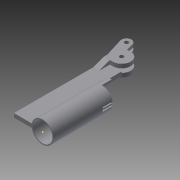
# Autodesk Inventor part: Base_Cylinder_1
Saved by Autodesk Inventor 2015 (Build 190159000, 159)
## iProperties
Created: 2016-07-06
Part Number: Base_Cylinder_1
Material: Generic
Document SubType Name: Modeling
Designer: Neelotpal Nag
Density: 1 g/cm^3
Appearance: Default
Mass: 1.76913 g
Surface Area: 37.308 cm^2
Volume: 1.76913 cm^3
Author: Neelotpal Nag
Autodesk Inventor part; units mm, degrees
ref_plane "YZ Plane" through (0, 0, 0) normal (1, 0, 0) x (0, 1, 0)
ref_plane "XZ Plane" through (0, 0, 0) normal (0, 1, 0) x (-1, 0, 0)
sketch "Sketch1" plane through (0, 0, 0) normal (0, 1, 0) x (-1, 0, 0)
  circle A0 centre (0, 0) radius 5
  circle A1 centre (0, 0) radius 5.5
  dimension "d0" = 10
  dimension "d1" = 11
  constraints: 2 centre point, 2 coincident
  measures "d0" diameter of A0
  measures "d1" diameter of A1
extrude "Extrusion1" add sketch "Sketch1" along normal blind 35
sketch "Sketch2" plane through (0, 0, 0) normal (0, 0, 1) x (1, 0, 0)
  point P0 (0, 0)
sketch "Sketch3" plane through (0, 0, 0) normal (0, 0, 1) x (1, 0, 0)
  line L0 (0, 0) -> (-10, 0)
  line L1 (-5.5, 0) -> (5.5, 0) projected
  circle A0 centre (-10, 50) radius 1
  line L2 (-5.5495, 50) -> (-5.5, 50)
  line L3 (-5.5, 50) -> (-5.5, 35)
  line L4 (5.5, 35) -> (-5.5, 35) projected
  line L5 (-14.5, 50) -> (-14.5, 0)
  line L6 (-14.5, 0) -> (-10, 0)
  circle A1 centre (-10, 50) radius 4.5
  line L7 (-10, 45.5) -> (-5.5, 45.5)
  line L8 (-14.5, 45.5) -> (-10, 45.5)
  line L9 (-5.5, 0) -> (-5.5, 50)
  line L10 (-5.5, 0) -> (-5.5, 45.5)
  line L11 (5, 0) -> (-5, 0) projected
  line L12 (-5.5, 0) -> (-5.5, 45.5)
  line L13 (-10, 0) -> (-5, 0)
  line L14 (-5.5, 45.5) -> (-5, 0)
  line L15 (-10, 0) -> (-10, 45.5)
  line L16 (-10, 45.5) -> (-5.5, 45.5)
  line L17 (-9, 50) -> (-10, 50)
  line L18 (-11, 50) -> (-14.5, 50)
  line L19 (-10, 0) -> (-10, 45.5)
  line L20 (-10, 49) -> (-10, 50)
  circle A2 centre (-10, 50) radius 4.5
  line L21 (-14.5, 45.5) -> (-14.5, 50)
  line L22 (-14.5, 45.5) -> (-5.5, 45.5)
  line L23 (-5.5, 45.5) -> (-5.5, 50)
  line L24 (-10, 50) -> (0, 50) construction
  line L25 (-10, 50) -> (-10.5736, 50.8192)
  circle A3 centre (-15.7358, 58.1915) radius 1
  circle A4 centre (-15.7358, 58.1915) radius 2.5
  point P0 (12.8857, 32.907)
  dimension "d4" = 10
  dimension "d5" = 50
  dimension "d7" = 2
  dimension "d8" = 9
  dimension "d19" = 2
  dimension "d20" = 5
  constraints: 47 end point, 8 collinear, 8 perpendicular, 7 coincident, 6 point on circle, 6 tangent, 5 centre point, 5 point on line, 2 horizontal, 2 vertical, 1 concentric
  measures "d4" distance of L0.start L0.end
  measures "d5" distance of L0.end L17.end
  measures "d7" diameter of A0
  measures "d8" distance of L2.end L5.start
  measures "d19" diameter of A3
  measures "d20" diameter of A4
extrude "Extrusion2" add sketch "Sketch3" along normal mid plane 2 contours L0 L9 L4 L14 | L0 L15 L7 L3 L9 | L4 L3 L14 | L6 L5 L8 L15
sketch "Sketch4" plane through (0, 0, 1) normal (0, 0, 1) x (1, 0, 0)
  circle A0 centre (-10, 50) radius 4.5 projected
  line L0 (-14.5, 50) -> (-14.5, 0) projected
  line L1 (-5.5, 50) -> (-5.5, 35) projected
  line L2 (-5.5, 45.5) -> (-14.5, 45.5) projected
  arc A1 (-14.5, 50) -> (-10, 45.5) centre (-10, 50) ccw
  line L3 (-10, 45.5) -> (-14.5, 45.5)
  line L4 (-14.5, 45.5) -> (-14.5, 50)
  point P0 (0, 0)
  constraints: 4 end point, 3 tangent, 2 point on circle, 1 centre point, 1 collinear, 1 concentric, 1 midpoint, 1 perpendicular
extrude "Extrusion3" add sketch "Sketch4" along normal blind 2 contours A0 L2 L0
sketch "Sketch5" plane through (0, 0, 1) normal (0, 0, 1) x (1, 0, 0)
  line L0 (-5.3846, 35) -> (-5.5, 45.5) projected
  line L1 (-5.4396, 40) -> (-14.5, 40)
  line L2 (-14.5, 45.5) -> (-14.5, 0) projected
  point P0 (0, 0)
  constraints: 2 end point, 2 point on line, 1 horizontal
sketch "Sketch6" plane through (-14.5, 45.5, 1) normal (-1, 0, 0) x (0, 0, 1)
  line L0 (2, 0) -> (0, -5.25)
  line L1 (0, -10.5) -> (0, 0) projected
  line L2 (2, 0) -> (0, 0)
  line L3 (0, 0) -> (0, -5.25)
  point P0 (-1, -45.5)
  constraints: 6 end point, 1 collinear, 1 horizontal, 1 midpoint
extrude "Extrusion4" add sketch "Sketch6" against normal blind 3
sketch "Sketch7" plane through (0, 0, 3) normal (0, 0, 1) x (1, 0, 0)
  circle A0 centre (-10, 50) radius 4.5 projected
  circle A1 centre (-10, 50) radius 1 projected
  point P0 (0, 0)
extrude "Extrusion5" add sketch "Sketch7" against normal blind 2
mirror "Mirror1" about plane through (0, 0, 0) normal (0, 0, 1) of "Extrusion4", "Extrusion3", "Extrusion5"
ref_plane "Work Plane1" through (0, 0, 0.75) normal (0, 0, 1) x (1, 0, 0)
sketch "Sketch8" plane through (0, 0, 0.75) normal (0, 0, 1) x (1, 0, 0)
  circle A0 centre (-15.7358, 58.1915) radius 2.5 projected
  circle A1 centre (-15.7358, 58.1915) radius 1 projected
  line L0 (-14.5, 45.5) -> (-18.1282, 57.4661)
  line L1 (-13.3433, 58.9169) -> (-12.1116, 53.9738)
  arc A2 (-10, 45.5) -> (-14.5, 50) centre (-10, 50) ccw projected
  arc A3 (-12.1116, 53.9738) -> (-14.5, 50) centre (-10, 50) ccw
  line L2 (-14.5, 45.5) -> (-14.5, 50)
  line L3 (-14.5, 50) -> (-14.5, 45.5) projected
  point P0 (0, 0)
  constraints: 6 end point, 5 point on circle, 1 centre point, 1 collinear, 1 concentric, 1 tangent
extrude "Extrusion6" add sketch "Sketch8" along normal blind 1.5
mirror "Mirror2" about plane through (0, 0, 0) normal (0, 0, 1) of "Extrusion6"
sketch "Sketch9" plane through (0, 0, 0) normal (0, 0, -1) x (1, 0, 0)
  point P0 (0, 0)
sketch "Sketch10" plane through (0, 35, 0) normal (0, 1, 0) x (1, 0, 0)
  line L0 (6.5, -1) -> (4.5, -1)
  line L1 (4.5, -1) -> (4.5, 1)
  line L2 (4.5, 1) -> (6.5, 1)
  line L3 (6.5, 1) -> (6.5, -1)
  arc A0 (-5.4083, -1) -> (-5.4083, 1) centre (0, 0) ccw projected
  line L4 (6.5, -1) -> (4.5, 1) construction
  line L5 (4.5, -1) -> (6.5, 1) construction
  point P0 (5.5, 0)
  dimension "d24" = 2
  dimension "d25" = 2
  constraints: 12 end point, 2 midpoint, 2 parallel, 1 horizontal, 1 perpendicular, 1 point on circle
  measures "d24" distance of L1.end L2.end
  measures "d25" distance of L0.end L1.end
extrude "Extrusion7" cut sketch "Sketch10" against normal blind 10
sketch "Sketch11" plane through (0, 35, 0) normal (0, 1, 0) x (1, 0, 0)
  line L0 (0, 5.5536) -> (9.1038, 5.5536)
  line L1 (9.1038, 5.5536) -> (9.1038, -5.5536)
  line L2 (9.1038, -5.5536) -> (0, -5.5536)
  line L3 (0, -5.5536) -> (0, 5.5536)
  point P0 (0, 0)
  constraints: 8 end point, 2 parallel, 1 horizontal, 1 perpendicular
extrude "Extrusion8" cut sketch "Sketch11" against normal blind 5
ref_plane "Work Plane2" through (0, 0, 0) normal (0, 0, 1) x (1, 0, 0)
body "Solid1"
